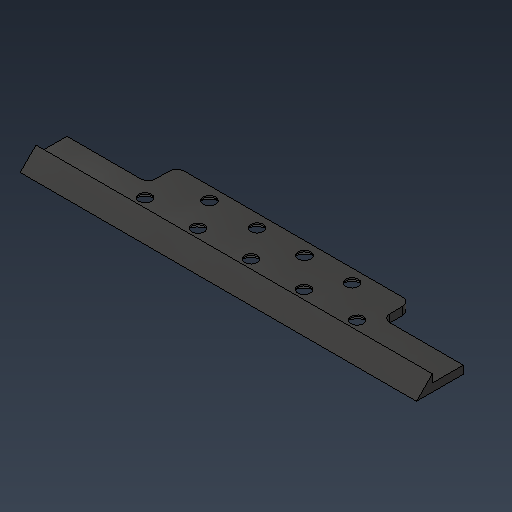
# Autodesk Inventor part: Plog2
Saved by Autodesk Inventor 2026.2 (Build 302298010, 298A)
## iProperties
Created: 2022-01-27
Part Number: Plog2
Material: Steel, Carbon
Document SubType Name: Modeling
Designer: Michał
Density: 7.85 g/cm^3
Appearance: Dark Gray
Mass: 23.2729 g
Surface Area: 39.2273 cm^2
Volume: 2.9647 cm^3
Author: Michał
Autodesk Inventor part; units mm, degrees
ref_plane "YZ Plane" through (0, 0, 0) normal (1, 0, 0) x (0, 1, 0)
ref_plane "XZ Plane" through (0, 0, 0) normal (0, 1, 0) x (-1, 0, 0)
ref_plane "XY Plane" through (0, 0, 0) normal (0, 0, 1) x (1, 0, 0)
sketch "Szkic1" plane through (0, 0, 0) normal (1, 0, 0) x (0, 1, 0)
  line L0 (0, 0) -> (2, -2)
  line L1 (2, -2) -> (2, -19)
  line L2 (2, -19) -> (0, -19)
  line L3 (0, -19) -> (0, -2)
  line L4 (0, -2) -> (0, 0)
  line L5 (0, -2) -> (2, -2)
  line L6 (2, -2) -> (4, -4)
  line L7 (4, -4) -> (2, -4)
  line L8 (2, -2) -> (4, -4)
  line L9 (4, -4) -> (2, -4)
  line L10 (4, -4) -> (4, -4)
  point P0 (5, -5)
  dimension "d1" = 2
  dimension "d2" = 45
  dimension "d44" = 45
  dimension "d45" = 2
  dimension "d46" = 17
  dimension "d50" = 4
  dimension "d51" = 19
  dimension "d54" = 0
  dimension "d98" = 2
  constraints: 22 end point, 6 perpendicular, 6 point on line, 1 vertical
  measures "d1" distance between parallel lines of L4 L1
  measures "d2" angle of L4 L0
  measures "d44" angle of L7 L6
  measures "d45" distance of L3.end L0.start
  measures "d46" distance of L2.end L3.end
  measures "d50" distance from line of L0.start L10
  measures "d51" distance from line of L2 L0.start
  measures "d54" distance from line of L10 L8.end
  measures "d98" distance from line of L1 L6.end
extrude "Wyciągnięcie proste1" add sketch "Szkic1" along normal mid plane 100
sketch "Sketch4" plane through (-50, 0, -19) normal (0, -1, 0) x (1, 0, 0)
  line L0 (0, 0) -> (0, 19) projected
  line L1 (0, 0) -> (100, 0) projected
  line L2 (100, 19) -> (100, 0) projected
  line L3 (100, 19) -> (0, 19) projected
  line L4 (80, 0) -> (80, 19)
  line L5 (100, 19) -> (50, 19) projected
  line L6 (20, 19) -> (20, 0)
  line L7 (0, 0) -> (100, 0) projected
  line L8 (0, 15) -> (100, 15) projected
  circle A0 centre (76.75, 10.75) radius 3.25
  circle A1 centre (63.375, 10.75) radius 3.25
  circle A2 centre (36.625, 10.75) radius 3.25
  circle A3 centre (23.25, 10.75) radius 3.25
  line L9 (80, 10.75) -> (20, 10.75)
  circle A4 centre (50, 10.75) radius 3.25
  circle A5 centre (68, 3.25) radius 3.25
  circle A6 centre (44, 3.25) radius 3.25
  circle A7 centre (32, 3.25) radius 3.25
  line L10 (80, 3.25) -> (20, 3.25)
  circle A8 centre (56, 3.25) radius 3.25
  dimension "d67" = 6.5
  dimension "d70" = 6.5
  dimension "d22" = 20
  dimension "d23" = 20
  dimension "d68" = 6.5
  dimension "d69" = 6.5
  dimension "d72" = 13.375
  dimension "d75" = 13.375
  dimension "d104" = 6.5
  dimension "d106" = 13.375
  dimension "d107" = 13.375
  dimension "d109" = 6.5
  dimension "d110" = 6.5
  dimension "d111" = 6.5
  dimension "d113" = 12
  dimension "d114" = 6.5
  dimension "d115" = 12
  dimension "d116" = 12
  dimension "d119" = 1
  dimension "d122" = 12
  dimension "d123" = 12
  dimension "d124" = 3.25
  constraints: 13 point on line, 8 end point, 7 centre point, 2 horizontal, 2 horizontal alignment, 2 perpendicular, 2 vertical, 1 midpoint, 4 other
  measures "d22" distance between parallel lines of L2 L4
  measures "d23" distance between parallel lines of L0 L6
  measures "d68" diameter of A1
  measures "d69" diameter of A2
  measures "d72" distance of A1.centre point (76.75, 10.75)
  measures "d75" distance of point (23.25, 10.75) A2.centre
  measures "d104" diameter of A4
  measures "d106" distance of A1.centre A4.centre
  measures "d107" distance of A2.centre A4.centre
  measures "d109" diameter of A5
  measures "d110" diameter of A6
  measures "d111" diameter of A7
  measures "d113" distance of A7.centre A6.centre
  measures "d114" diameter of A8
  measures "d115" distance of A5.centre A8.centre
  measures "d116" distance of A6.centre A8.centre
  measures "d122" distance from line of A5.centre L4
  measures "d123" distance from line of L6 A7.centre
  measures "d124" distance from line of A5.centre L1
hole "Hole2" at (26.75, 0, -8.25) at (13.375, 0, -8.25) at (-13.375, 0, -8.25) at (-26.75, 0, -8.25) at (0, 0, -8.25) at (-18, 0, -15.75) at (-6, 0, -15.75) at (6, 0, -15.75) at (18, 0, -15.75) direction (0, 1, 0) diameter 3.2 depth 8.8 countersink diameter 6.5 countersink angle 90 clearance for "Countersunk Flat Head Screw ISO 2009/7046" size "M3" standard "ISO"
sketch "Sketch5" plane through (-50, 0, 0) normal (0, -1, 0) x (1, 0, 0)
  line L0 (100, 0) -> (100, -19) projected
  line L1 (100, 0) -> (0, 0) projected
  line L2 (0, -19) -> (0, 0) projected
  line L3 (100, -11.808) -> (79.5, -11.808)
  line L4 (79.5, -11.808) -> (79.5, -28.94)
  line L5 (79.5, -28.94) -> (100, -28.94)
  line L6 (100, -28.94) -> (100, -11.808)
  line L7 (0, -19) -> (20.5, -19)
  line L8 (20.5, -19) -> (20.5, -11.808)
  line L9 (20.5, -11.808) -> (0, -11.808)
  line L10 (0, -11.808) -> (0, -19)
  circle A0 centre (23.25, -8.25) radius 3.25 projected
  circle A1 centre (36.625, -8.25) radius 3.25 projected
  circle A2 centre (63.375, -8.25) radius 3.25 projected
  circle A3 centre (76.75, -8.25) radius 3.25 projected
  line L11 (68, -19) -> (100, -19) projected
  circle A4 centre (50, -8.25) radius 3.25 projected
  circle A5 centre (56, -15.75) radius 3.25 projected
  circle A6 centre (44, -15.75) radius 3.25 projected
  circle A7 centre (68, -15.75) radius 3.25 projected
  circle A8 centre (32, -15.75) radius 3.25 projected
  line L12 (0, -19) -> (32, -19) projected
  line L13 (32, -19) -> (44, -19) projected
  line L14 (44, -19) -> (56, -19) projected
  line L15 (56, -19) -> (68, -19) projected
  point P0 (50, 0)
  point P1 (0, -11.808)
  point P2 (100, -30)
  point P3 (20, -19)
  point P4 (20, -19)
  point P5 (79.5, -19)
  dimension "d55" = 20.5
  dimension "d56" = 20.5
  dimension "d61" = 11.808
  dimension "d62" = 11.808
  constraints: 16 end point, 4 parallel, 4 vertical alignment, 2 horizontal, 2 perpendicular, 1 point on line
  measures "d55" distance of L8.end L9.end
  measures "d56" distance of L3.start L3.end
  measures "d61" distance between parallel lines of L1 L9
  measures "d62" distance between parallel lines of L1 L3
extrude "Extrusion5" cut sketch "Sketch5" against normal through all contours L0 L11 L4 L3 | L6 L5 L4 L11 | L9 L8 L7 L2
fillet "Fillet2" radius 2 4 edges at (29.5, 1, -11.808) (-29.5, 1, -11.808) (-29.5, 1, -19) (29.5, 1, -19)
equation "\"d23\" = d22"
equation "\"d72\" = d75"
equation "\"d56\" = d55"
equation "\"d62\" = d61"
equation "\"d64\" = d80"
equation "\"d79\" = d64"
equation "\"d80\" = 4.648267"
